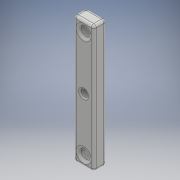
# Autodesk Inventor part: 핸들
Saved by Autodesk Inventor 2018 (Build 220112000, 112)
## iProperties
Created: 2019-11-05
Part Number: 핸들
Material: 일반
Document SubType Name: Modeling
Designer: LeeYounSeo
Density: 1 g/cm^3
Appearance: 기본값
Author: LeeYounSeo
Autodesk Inventor part; units mm, degrees
ref_plane "YZ Plane" through (0, 0, 0) normal (1, 0, 0) x (0, 1, 0)
ref_plane "XZ Plane" through (0, 0, 0) normal (0, 1, 0) x (-1, 0, 0)
ref_plane "XY Plane" through (0, 0, 0) normal (0, 0, 1) x (1, 0, 0)
sketch "스케치1" plane through (0, 0, 0) normal (0, 1, 0) x (-1, 0, 0)
  line L0 (0, 0) -> (8, 0)
  line L1 (8, 0) -> (8, -50)
  line L2 (8, -50) -> (0, -50)
  line L3 (0, -50) -> (0, 0)
  dimension "d0" = 50
  dimension "d1" = 8
  constraints: 8 end point, 2 parallel, 1 horizontal, 1 perpendicular
  measures "d0" distance of L0.end L1.end
  measures "d1" distance of L1.end L2.end
extrude "돌출1" add sketch "스케치1" along normal blind 5
sketch "스케치2" plane through (0, 5, 0) normal (0, 1, 0) x (1, 0, 0)
  circle A0 centre (-4, 4) radius 2
  line L0 (-8, 50) -> (-8, 0) projected
  line L1 (-8, 0) -> (0, 0) projected
  circle A1 centre (-4, 46) radius 2
  line L2 (0, 0) -> (0, 50) projected
  line L3 (0, 50) -> (-8, 50) projected
  dimension "d4" = 4
  dimension "d5" = 4
  dimension "d6" = 4
  dimension "d7" = 4
  dimension "d8" = 4
  dimension "d9" = 4
  constraints: 2 centre point
  measures "d4" diameter of A0
  measures "d5" distance from line of L0 A0.centre
  measures "d6" distance from line of A0.centre L1
  measures "d7" diameter of A1
  measures "d8" distance from line of L2 A1.centre
  measures "d9" distance from line of L3 A1.centre
sketch "스케치3" plane through (0, 0, 0) normal (0, -1, 0) x (1, 0, 0)
  circle A0 centre (-4, -25) radius 1.5
  line L0 (-8, -50) -> (0, -50) projected
  line L1 (0, -50) -> (0, 0) projected
  dimension "d10" = 3
  dimension "d11" = 25
  dimension "d12" = 4
  constraints: 1 centre point
  measures "d10" diameter of A0
  measures "d11" distance from line of L0 A0.centre
  measures "d12" distance from line of L1 A0.centre
extrude "돌출2" cut sketch "스케치2" against normal blind 5 contours A0 | A1
extrude "돌출3" cut sketch "스케치3" against normal blind 5
fillet "모깎기1" radius 1 12 edges at (-8, 5, -25) (-4, 5, 0) (0, 5, -25) (-4, 0, 0) (0, 0, -25) (0, 2.5, 0) (-8, 2.5, 0) (0, 2.5, -50) (-4, 5, -50) (-4, 0, -50) (-8, 2.5, -50) (-8, 0, -25)
fillet "모깎기2" radius 0.5 1 edges at (-5.5, 0, -25)
fillet "모깎기3" radius 1 4 edges at (-6, 0, -46) (-6, 0, -4) (-6, 5, -4) (-6, 5, -46)
